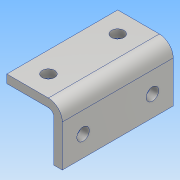
# Autodesk Inventor part: Timing_Angle Bracket
Saved by Autodesk Inventor 2018.1 (Build 221171000, 171)
## iProperties
Created: 2019-02-12
Part Number: Timing_Angle Bracket
Material: Aluminum 6061
Document SubType Name: Modeling
Designer: James
Density: 2.7 g/cm^3
Appearance: Aluminum - Flat
Author: James
Autodesk Inventor part; units mm, degrees
ref_plane "YZ Plane" through (0, 0, 0) normal (1, 0, 0) x (0, 1, 0)
ref_plane "XZ Plane" through (0, 0, 0) normal (0, 1, 0) x (-1, 0, 0)
ref_plane "XY Plane" through (0, 0, 0) normal (0, 0, 1) x (1, 0, 0)
sketch "Sketch1" plane through (0, 0, 0) normal (0, 1, 0) x (-1, 0, 0)
  line L0 (0, 0) -> (20, 0)
  line L1 (20, 0) -> (20, -3)
  line L2 (20, -3) -> (0, -3)
  line L3 (0, -3) -> (0, 0)
  line L4 (0, 0) -> (3, 0)
  line L5 (3, 0) -> (3, -20)
  line L6 (3, -20) -> (0, -20)
  line L7 (0, -20) -> (0, 0)
  dimension "d0" = 3
  dimension "d1" = 3
  dimension "d2" = 20
  dimension "d3" = 20
  constraints: 16 end point, 4 parallel, 2 horizontal, 2 perpendicular
  measures "d0" distance of L5.end L6.end
  measures "d1" distance of L0.end L1.end
  measures "d2" distance of L0.start L0.end
  measures "d3" distance of L6.end L0.start
extrude "Extrusion1" add sketch "Sketch1" along normal blind 40
fillet "Fillet1" radius 2 1 edges at (-3, 20, -3)
fillet "Fillet2" radius 5 1 edges at (0, 20, 0)
sketch "Sketch2" plane through (-3, 0, -20) normal (-1, 0, 0) x (0, 0, 1)
  line L0 (0, 40) -> (15, 40) projected
  line L1 (0, 0) -> (15, 0) projected
  line L2 (0, 0) -> (0, 40) projected
  point P0 (20, 0)
  point P1 (7.5, 32.5)
  point P2 (7.5, 7.5)
  dimension "d8" = 7.5
  dimension "d9" = 7.5
  dimension "d10" = 25
  dimension "d11" = 7.5
  constraints: 1 vertical alignment
  measures "d8" distance from line of L0 point (7.5, 32.5)
  measures "d9" distance from line of L1 point (7.5, 7.5)
  measures "d10" distance of point (7.5, 32.5) point (7.5, 7.5)
  measures "d11" distance from line of L2 point (7.5, 32.5)
hole "Hole1" at (-3, 32.5, -12.5) at (-3, 7.5, -12.5) direction (1, 0, 0) diameter 4.5 end through all clearance for "Socket Head Cap Screw" size "M4" standard "Ansi Metric M Profile"
sketch "Sketch3" plane through (-20, 0, -3) normal (0, 0, -1) x (-1, 0, 0)
  line L0 (-15, 40) -> (0, 40) projected
  line L1 (-15, 0) -> (0, 0) projected
  line L2 (0, 0) -> (0, 40) projected
  point P0 (-20, 0)
  point P1 (-7.5, 32.5)
  point P2 (-7.5, 7.5)
  dimension "d19" = 7.5
  dimension "d20" = 7.5
  dimension "d21" = 7.5
  constraints: 1 vertical alignment
  measures "d19" distance from line of L0 point (-7.5, 32.5)
  measures "d20" distance from line of L1 point (-7.5, 7.5)
  measures "d21" distance from line of L2 point (-7.5, 32.5)
hole "Hole2" at (-12.5, 32.5, -3) at (-12.5, 7.5, -3) direction (0, 0, 1) diameter 4.5 end through all clearance for "Socket Head Cap Screw" size "M4" standard "Ansi Metric M Profile"
equation "\"d1\" = d0"
equation "\"d3\" = d2"
equation "\"d9\" = d8"
equation "\"d20\" = d19"
equation "\"d21\" = d19"
body "Solid1"
